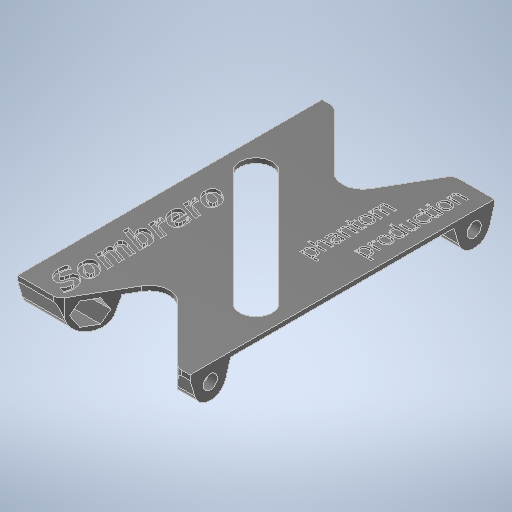
# Autodesk Inventor part: 3D_side-wall
Saved by Autodesk Inventor 2025 (Build 290162000, 162)
## iProperties
Created: 2024-06-30
Part Number: 3D_side-wall
Material: 一般
Document SubType Name: Modeling
Designer: 8326d
Density: 1 g/cm^3
Appearance: 滑らか - 黒
Author: 8326d
## iProperties of the stored document 3D_side-wall_3D プリント.ipt
Created: 2024-07-25
Part Number: 3D_side-wall_3D プリント
Material: 一般
Document SubType Name: Modeling
Designer: 8326d
Density: 1 g/cm^3
Appearance: 既定
Author: 8326d
Autodesk Inventor part; units mm, degrees
ref_plane "YZ Plane" through (0, 0, 0) normal (1, 0, 0) x (0, 1, 0)
ref_plane "XZ Plane" through (0, 0, 0) normal (0, 1, 0) x (-1, 0, 0)
ref_plane "XY Plane" through (0, 0, 0) normal (0, 0, 1) x (1, 0, 0)
sketch "スケッチ1" plane through (0, 0, 0) normal (0, 1, 0) x (-1, 0, 0)
  line L0 (-21.25, 37.5) -> (21.25, 37.5)
  line L1 (21.25, 37.5) -> (21.25, -37.5)
  line L2 (21.25, -37.5) -> (-21.25, -37.5)
  line L3 (-21.25, -37.5) -> (-21.25, 37.5)
  line L4 (-21.25, 37.5) -> (21.25, -37.5) construction
  line L5 (21.25, 37.5) -> (-21.25, -37.5) construction
  point P0 (0, 0)
  dimension "d0" = 42.5
  dimension "d1" = 75
  constraints: 12 end point, 2 midpoint, 2 parallel, 1 horizontal, 1 perpendicular
  measures "d0" distance of L1.end L2.end
  measures "d1" distance of L0.end L1.end
extrude "押し出し1" add sketch "スケッチ1" along normal mid plane 1.2
sketch "スケッチ2" plane through (21.25, 0.6, 37.5) normal (1, 0, 0) x (0, 0, -1)
  line L0 (0, 0) -> (75, 0) projected
  circle A0 centre (5, -4) radius 4
  line L1 (75, 0) -> (0, 0) projected
  circle A1 centre (70, -4) radius 4
  line L2 (75, -1.2) -> (0, -1.2) projected
  line L3 (1.1644, -5.135) -> (0, -1.2)
  line L4 (8.8356, -5.135) -> (10, -1.2)
  line L5 (66.1644, -5.135) -> (65, -1.2)
  line L6 (0, -1.2) -> (75, -1.2) projected
  line L7 (73.8356, -5.135) -> (75, -1.2)
  point P0 (37.5, -0.6)
  point P1 (67.1434, -1.2)
  point P2 (72.8566, -1.2)
  point P3 (2.1434, -1.2)
  point P4 (7.8566, -1.2)
  dimension "d4" = 8
  dimension "d5" = 8
  dimension "d6" = 5
  dimension "d7" = 5
  dimension "d8" = 5
  dimension "d9" = 5
  constraints: 8 end point, 6 tangent, 4 point on circle, 2 centre point, 2 point on line
  measures "d4" diameter of A0
  measures "d5" diameter of A1
  measures "d6" horizontal distance of L0.start A0.centre
  measures "d7" horizontal distance of L0.end A1.centre
  measures "d8" horizontal distance of A1.centre L5.end
  measures "d9" horizontal distance of A0.centre L4.end
extrude "押し出し2" add sketch "スケッチ2" against normal up to surface (42.5 mm away) contours A0 L2 | A1 L2 | L2 L4 A0 | A0 L2 | A0 L3 L2 | L2 L7 A1 | A1 L2 | A1 L5 L2
sketch "スケッチ3" plane through (0, 0.6, 0) normal (0, 1, 0) x (1, 0, 0)
  line L0 (14.1421, -14.1421) -> (-14.1421, 14.1421) construction
  line L1 (16.9706, -11.3137) -> (-11.3137, 16.9706)
  line L2 (-16.9706, 11.3137) -> (11.3137, -16.9706)
  arc A0 (11.3137, -16.9706) -> (16.9706, -11.3137) centre (14.1421, -14.1421) ccw
  arc A1 (-11.3137, 16.9706) -> (-16.9706, 11.3137) centre (-14.1421, 14.1421) ccw
  line L3 (-21.25, 37.5) -> (-21.25, -37.5) projected
  point P0 (0, 0)
  dimension "d12" = 45
  dimension "d13" = 40
  dimension "d14" = 4
  constraints: 8 end point, 4 point on circle, 4 tangent, 2 centre point, 1 midpoint, 1 parallel
  measures "d12" angle of L3 L0
  measures "d13" distance of L0.start L0.end
  measures "d14" radius of A1
extrude "押し出し3" cut sketch "スケッチ3" against normal through all
sketch "スケッチ4" plane through (0, 0.6, 0) normal (0, 1, 0) x (1, 0, 0)
  line L0 (7.2681, 1.9828) -> (7.2681, 38.4533) construction
  line L1 (7.2681, 38.4533) -> (15.699, 38.4533) construction
  line L2 (15.699, 38.4533) -> (15.699, 1.9828) construction
  line L3 (15.699, 1.9828) -> (7.2681, 1.9828) construction
  line L4 (-17.7945, -35.8694) -> (-17.7945, 8.3303) construction
  line L5 (-17.7945, 8.3303) -> (-9.6917, 8.3303) construction
  line L6 (-9.6917, 8.3303) -> (-9.6917, -35.8694) construction
  line L7 (-9.6917, -35.8694) -> (-17.7945, -35.8694) construction
  spline S0 degree 2 poles (-11.4201, -33.4285) (-11.4201, -34.119) (-11.6875, -35.072) (-11.882, -35.4512) knots 0 0 0 1 2 2 2
  line L8 (-11.882, -35.4512) -> (-13.3115, -34.965)
  line L9 (-13.3115, -34.965) -> (-13.3115, -34.8289)
  spline S1 degree 2 poles (-13.3115, -34.8289) (-12.9274, -34.508) (-12.5141, -33.5647) (-12.5141, -33.0541) knots 0 0 0 1 2 2 2
  spline S2 degree 2 poles (-12.5141, -33.0541) (-12.5141, -32.9229) (-12.5725, -32.4804) (-12.6308, -32.3345) knots 0 0 0 1 2 2 2
  spline S3 degree 2 poles (-12.6308, -32.3345) (-12.6989, -32.1546) (-12.9469, -31.8532) (-13.1462, -31.7851) knots 0 0 0 1 2 2 2
  spline S4 degree 2 poles (-13.1462, -31.7851) (-13.3747, -31.7073) (-13.6568, -31.965) (-13.72, -32.1887) knots 0 0 0 1 2 2 2
  spline S5 degree 2 poles (-13.72, -32.1887) (-13.8026, -32.4658) (-13.9436, -33.1125) (-14.0506, -33.3799) knots 0 0 0 1 2 2 2
  spline S6 degree 2 poles (-14.0506, -33.3799) (-14.2937, -33.9926) (-15.1252, -34.3183) (-15.7475, -34.1044) knots 0 0 0 1 2 2 2
  spline S7 degree 2 poles (-15.7475, -34.1044) (-16.5887, -33.8175) (-17.6341, -32.0379) (-17.6341, -30.9683) knots 0 0 0 1 2 2 2
  spline S8 degree 2 poles (-17.6341, -30.9683) (-17.6341, -30.4334) (-17.4153, -29.4512) (-17.2305, -29.0914) knots 0 0 0 1 2 2 2
  line L10 (-17.2305, -29.0914) -> (-15.8593, -29.5582)
  line L11 (-15.8593, -29.5582) -> (-15.8593, -29.6943)
  spline S9 degree 2 poles (-15.8593, -29.6943) (-16.1462, -29.9277) (-16.5401, -30.7543) (-16.5401, -31.2648) knots 0 0 0 1 2 2 2
  spline S10 degree 2 poles (-16.5401, -31.2648) (-16.5401, -31.4593) (-16.4817, -31.7948) (-16.4039, -31.9942) knots 0 0 0 1 2 2 2
  spline S11 degree 2 poles (-16.4039, -31.9942) (-16.3407, -32.1546) (-16.0879, -32.4464) (-15.9323, -32.4999) knots 0 0 0 1 2 2 2
  spline S12 degree 2 poles (-15.9323, -32.4999) (-15.6989, -32.5777) (-15.4315, -32.3443) (-15.3245, -31.9164) knots 0 0 0 1 2 2 2
  spline S13 degree 2 poles (-15.3245, -31.9164) (-15.2564, -31.6344) (-15.1252, -31.119) (-15.0133, -30.8418) knots 0 0 0 1 2 2 2
  spline S14 degree 2 poles (-15.0133, -30.8418) (-14.7848, -30.2924) (-14.0263, -29.9423) (-13.4039, -30.1563) knots 0 0 0 1 2 2 2
  spline S15 degree 2 poles (-13.4039, -30.1563) (-12.5093, -30.4577) (-11.4201, -32.2324) (-11.4201, -33.4285) knots 0 0 0 1 2 2 2
  spline S16 degree 2 poles (-13.788, -24.9926) (-12.6697, -25.3718) (-11.3861, -27.0298) (-11.3861, -28.1433) knots 0 0 0 1 2 2 2
  spline S17 degree 2 poles (-11.3861, -28.1433) (-11.3861, -29.2519) (-12.6697, -30.0444) (-13.788, -29.6652) knots 0 0 0 1 2 2 2
  spline S18 degree 2 poles (-13.788, -29.6652) (-14.9161, -29.2811) (-16.1948, -27.6182) (-16.1948, -26.5096) knots 0 0 0 1 2 2 2
  spline S19 degree 2 poles (-16.1948, -26.5096) (-16.1948, -25.401) (-14.9112, -24.6133) (-13.788, -24.9926) knots 0 0 0 1 2 2 2
  spline S20 degree 2 poles (-13.7783, -26.4415) (-14.1819, -26.3005) (-14.7216, -26.2519) (-14.882, -26.3151) knots 0 0 0 1 2 2 2
  spline S21 degree 2 poles (-14.882, -26.3151) (-15.0522, -26.3832) (-15.1835, -26.6506) (-15.1835, -26.8548) knots 0 0 0 1 2 2 2
  spline S22 degree 2 poles (-15.1835, -26.8548) (-15.1835, -27.0444) (-15.0668, -27.3896) (-14.9015, -27.5744) knots 0 0 0 1 2 2 2
  spline S23 degree 2 poles (-14.9015, -27.5744) (-14.7459, -27.7494) (-14.1965, -28.0801) (-13.7783, -28.2259) knots 0 0 0 1 2 2 2
  spline S24 degree 2 poles (-13.7783, -28.2259) (-13.365, -28.367) (-12.8545, -28.401) (-12.6989, -28.3426) knots 0 0 0 1 2 2 2
  spline S25 degree 2 poles (-12.6989, -28.3426) (-12.5433, -28.2843) (-12.3974, -27.9974) (-12.3974, -27.7883) knots 0 0 0 1 2 2 2
  spline S26 degree 2 poles (-12.3974, -27.7883) (-12.3974, -27.6182) (-12.5433, -27.2195) (-12.6892, -27.0639) knots 0 0 0 1 2 2 2
  spline S27 degree 2 poles (-12.6892, -27.0639) (-12.8593, -26.8791) (-13.3504, -26.5874) (-13.7783, -26.4415) knots 0 0 0 1 2 2 2
  line L12 (-11.5271, -19.6101) -> (-13.788, -18.8418)
  spline S28 degree 2 poles (-13.788, -18.8418) (-14.1235, -18.73) (-14.5806, -18.5987) (-14.7264, -18.6084) knots 0 0 0 1 2 2 2
  spline S29 degree 2 poles (-14.7264, -18.6084) (-14.8723, -18.6182) (-15.0036, -18.8272) (-15.0036, -19.0558) knots 0 0 0 1 2 2 2
  spline S30 degree 2 poles (-15.0036, -19.0558) (-15.0036, -19.2162) (-14.8626, -19.576) (-14.7313, -19.8046) knots 0 0 0 1 2 2 2
  line L13 (-14.7313, -19.8046) -> (-11.5271, -20.8937)
  line L14 (-11.5271, -20.8937) -> (-11.5271, -22.3135)
  line L15 (-11.5271, -22.3135) -> (-13.788, -21.5452)
  spline S31 degree 2 poles (-13.788, -21.5452) (-14.1187, -21.4334) (-14.5806, -21.3021) (-14.7264, -21.3167) knots 0 0 0 1 2 2 2
  spline S32 degree 2 poles (-14.7264, -21.3167) (-14.8723, -21.3264) (-15.0036, -21.5355) (-15.0036, -21.764) knots 0 0 0 1 2 2 2
  spline S33 degree 2 poles (-15.0036, -21.764) (-15.0036, -21.9342) (-14.8431, -22.3232) (-14.7313, -22.5177) knots 0 0 0 1 2 2 2
  line L16 (-14.7313, -22.5177) -> (-11.5271, -23.6068)
  line L17 (-11.5271, -23.6068) -> (-11.5271, -25.0169)
  line L18 (-11.5271, -25.0169) -> (-16.0538, -23.4804)
  line L19 (-16.0538, -23.4804) -> (-16.0538, -22.0704)
  line L20 (-16.0538, -22.0704) -> (-15.553, -22.2405)
  spline S34 degree 2 poles (-15.553, -22.2405) (-15.8448, -21.7932) (-16.1754, -21.0639) (-16.1754, -20.6846) knots 0 0 0 1 2 2 2
  spline S35 degree 2 poles (-16.1754, -20.6846) (-16.1754, -20.2665) (-15.7816, -19.7705) (-15.3877, -19.7365) knots 0 0 0 1 2 2 2
  spline S36 degree 2 poles (-15.3877, -19.7365) (-15.767, -19.2016) (-16.1754, -18.3459) (-16.1754, -17.9764) knots 0 0 0 1 2 2 2
  spline S37 degree 2 poles (-16.1754, -17.9764) (-16.1754, -17.6603) (-15.976, -17.2324) (-15.7718, -17.1255) knots 0 0 0 1 2 2 2
  spline S38 degree 2 poles (-15.7718, -17.1255) (-15.553, -17.0088) (-14.955, -17.0234) (-14.4736, -17.1887) knots 0 0 0 1 2 2 2
  line L21 (-14.4736, -17.1887) -> (-11.5271, -18.1903)
  line L22 (-11.5271, -18.1903) -> (-11.5271, -19.6101)
  spline S39 degree 2 poles (-13.8512, -11.9229) (-12.7718, -12.2875) (-11.4396, -13.8337) (-11.4396, -14.6457) knots 0 0 0 1 2 2 2
  spline S40 degree 2 poles (-11.4396, -14.6457) (-11.4396, -14.9812) (-11.5903, -15.4334) (-11.7508, -15.6571) knots 0 0 0 1 2 2 2
  line L23 (-11.7508, -15.6571) -> (-11.5271, -15.7932)
  line L24 (-11.5271, -15.7932) -> (-11.5271, -17.1449)
  line L25 (-11.5271, -17.1449) -> (-17.7945, -15.0153)
  line L26 (-17.7945, -15.0153) -> (-17.7945, -13.6052)
  line L27 (-17.7945, -13.6052) -> (-15.5773, -14.3588)
  spline S41 degree 2 poles (-15.5773, -14.3588) (-15.8448, -13.9553) (-16.1754, -13.2016) (-16.1754, -12.7786) knots 0 0 0 1 2 2 2
  spline S42 degree 2 poles (-16.1754, -12.7786) (-16.1754, -11.9909) (-14.9452, -11.5485) (-13.8512, -11.9229) knots 0 0 0 1 2 2 2
  spline S43 degree 2 poles (-13.8221, -13.3767) (-14.4979, -13.1433) (-15.0765, -13.3572) (-15.0765, -13.7851) knots 0 0 0 1 2 2 2
  spline S44 degree 2 poles (-15.0765, -13.7851) (-15.0765, -13.9747) (-14.955, -14.388) (-14.8334, -14.6117) knots 0 0 0 1 2 2 2
  line L28 (-14.8334, -14.6117) -> (-12.5676, -15.3799)
  spline S45 degree 2 poles (-12.5676, -15.3799) (-12.5093, -15.2584) (-12.4704, -14.9861) (-12.4704, -14.8451) knots 0 0 0 1 2 2 2
  spline S46 degree 2 poles (-12.4704, -14.8451) (-12.4704, -14.3345) (-13.1462, -13.6052) (-13.8221, -13.3767) knots 0 0 0 1 2 2 2
  line L29 (-14.7167, -7.8094) -> (-14.7167, -7.9261)
  spline S47 degree 2 poles (-14.7167, -7.9261) (-14.7459, -7.999) (-14.7751, -8.2956) (-14.7751, -8.4804) knots 0 0 0 1 2 2 2
  spline S48 degree 2 poles (-14.7751, -8.4804) (-14.7751, -8.6992) (-14.6438, -9.2341) (-14.5563, -9.4917) knots 0 0 0 1 2 2 2
  line L30 (-14.5563, -9.4917) -> (-11.5271, -10.5225)
  line L31 (-11.5271, -10.5225) -> (-11.5271, -11.9326)
  line L32 (-11.5271, -11.9326) -> (-16.0538, -10.3961)
  line L33 (-16.0538, -10.3961) -> (-16.0538, -8.9861)
  line L34 (-16.0538, -8.9861) -> (-15.4023, -9.2049)
  spline S49 degree 2 poles (-15.4023, -9.2049) (-15.4898, -9.0785) (-15.7621, -8.6457) (-15.8448, -8.4755) knots 0 0 0 1 2 2 2
  spline S50 degree 2 poles (-15.8448, -8.4755) (-15.9371, -8.2908) (-16.0684, -7.8386) (-16.0684, -7.6587) knots 0 0 0 1 2 2 2
  spline S51 degree 2 poles (-16.0684, -7.6587) (-16.0684, -7.5858) (-16.0587, -7.4204) (-16.0538, -7.3572) knots 0 0 0 1 2 2 2
  line L35 (-16.0538, -7.3572) -> (-14.7167, -7.8094)
  spline S52 degree 2 poles (-11.4055, -6.0785) (-11.4055, -7.3621) (-12.6308, -8.3102) (-13.7637, -7.9261) knots 0 0 0 1 2 2 2
  spline S53 degree 2 poles (-13.7637, -7.9261) (-14.8723, -7.5469) (-16.1948, -5.8256) (-16.1948, -4.6781) knots 0 0 0 1 2 2 2
  spline S54 degree 2 poles (-16.1948, -4.6781) (-16.1948, -3.6376) (-15.0717, -2.9715) (-14.0311, -3.3264) knots 0 0 0 1 2 2 2
  line L36 (-14.0311, -3.3264) -> (-13.5206, -3.5015)
  line L37 (-13.5206, -3.5015) -> (-13.5206, -6.5987)
  spline S55 degree 2 poles (-13.5206, -6.5987) (-13.2046, -6.6814) (-12.7864, -6.5987) (-12.66, -6.4577) knots 0 0 0 1 2 2 2
  spline S56 degree 2 poles (-12.66, -6.4577) (-12.5336, -6.3167) (-12.4266, -5.8694) (-12.4266, -5.5825) knots 0 0 0 1 2 2 2
  spline S57 degree 2 poles (-12.4266, -5.5825) (-12.4266, -5.3394) (-12.5336, -4.824) (-12.626, -4.5955) knots 0 0 0 1 2 2 2
  spline S58 degree 2 poles (-12.626, -4.5955) (-12.6989, -4.3961) (-12.8788, -4.0412) (-12.9469, -3.9245) knots 0 0 0 1 2 2 2
  line L38 (-12.9469, -3.9245) -> (-12.9469, -3.7786)
  line L39 (-12.9469, -3.7786) -> (-11.7799, -4.1725)
  spline S59 degree 2 poles (-11.7799, -4.1725) (-11.7119, -4.3718) (-11.5952, -4.6976) (-11.5368, -4.965) knots 0 0 0 1 2 2 2
  spline S60 degree 2 poles (-11.5368, -4.965) (-11.4736, -5.2178) (-11.4055, -5.7284) (-11.4055, -6.0785) knots 0 0 0 1 2 2 2
  spline S61 degree 2 poles (-14.3715, -4.6003) (-14.8188, -4.4593) (-15.2905, -4.6927) (-15.2905, -5.0963) knots 0 0 0 1 2 2 2
  spline S62 degree 2 poles (-15.2905, -5.0963) (-15.2905, -5.5096) (-14.7945, -6.1417) (-14.3715, -6.3118) knots 0 0 0 1 2 2 2
  line L40 (-14.3715, -6.3118) -> (-14.3715, -4.6003)
  line L41 (-14.7167, 0.6703) -> (-14.7167, 0.5536)
  spline S63 degree 2 poles (-14.7167, 0.5536) (-14.7459, 0.4807) (-14.7751, 0.1841) (-14.7751, -0.0007) knots 0 0 0 1 2 2 2
  spline S64 degree 2 poles (-14.7751, -0.0007) (-14.7751, -0.2195) (-14.6438, -0.7543) (-14.5563, -1.012) knots 0 0 0 1 2 2 2
  line L42 (-14.5563, -1.012) -> (-11.5271, -2.0428)
  line L43 (-11.5271, -2.0428) -> (-11.5271, -3.4529)
  line L44 (-11.5271, -3.4529) -> (-16.0538, -1.9164)
  line L45 (-16.0538, -1.9164) -> (-16.0538, -0.5063)
  line L46 (-16.0538, -0.5063) -> (-15.4023, -0.7251)
  spline S65 degree 2 poles (-15.4023, -0.7251) (-15.4898, -0.5987) (-15.7621, -0.166) (-15.8448, 0.0042) knots 0 0 0 1 2 2 2
  spline S66 degree 2 poles (-15.8448, 0.0042) (-15.9371, 0.189) (-16.0684, 0.6412) (-16.0684, 0.8211) knots 0 0 0 1 2 2 2
  spline S67 degree 2 poles (-16.0684, 0.8211) (-16.0684, 0.894) (-16.0587, 1.0593) (-16.0538, 1.1225) knots 0 0 0 1 2 2 2
  line L47 (-16.0538, 1.1225) -> (-14.7167, 0.6703)
  spline S68 degree 2 poles (-13.788, 5.236) (-12.6697, 4.8567) (-11.3861, 3.1987) (-11.3861, 2.0852) knots 0 0 0 1 2 2 2
  spline S69 degree 2 poles (-11.3861, 2.0852) (-11.3861, 0.9766) (-12.6697, 0.1841) (-13.788, 0.5634) knots 0 0 0 1 2 2 2
  spline S70 degree 2 poles (-13.788, 0.5634) (-14.9161, 0.9475) (-16.1948, 2.6104) (-16.1948, 3.7189) knots 0 0 0 1 2 2 2
  spline S71 degree 2 poles (-16.1948, 3.7189) (-16.1948, 4.8275) (-14.9112, 5.6152) (-13.788, 5.236) knots 0 0 0 1 2 2 2
  spline S72 degree 2 poles (-13.7783, 3.787) (-14.1819, 3.928) (-14.7216, 3.9766) (-14.882, 3.9134) knots 0 0 0 1 2 2 2
  spline S73 degree 2 poles (-14.882, 3.9134) (-15.0522, 3.8454) (-15.1835, 3.5779) (-15.1835, 3.3737) knots 0 0 0 1 2 2 2
  spline S74 degree 2 poles (-15.1835, 3.3737) (-15.1835, 3.1841) (-15.0668, 2.8389) (-14.9015, 2.6541) knots 0 0 0 1 2 2 2
  spline S75 degree 2 poles (-14.9015, 2.6541) (-14.7459, 2.4791) (-14.1965, 2.1484) (-13.7783, 2.0026) knots 0 0 0 1 2 2 2
  spline S76 degree 2 poles (-13.7783, 2.0026) (-13.365, 1.8616) (-12.8545, 1.8275) (-12.6989, 1.8859) knots 0 0 0 1 2 2 2
  spline S77 degree 2 poles (-12.6989, 1.8859) (-12.5433, 1.9442) (-12.3974, 2.2311) (-12.3974, 2.4402) knots 0 0 0 1 2 2 2
  spline S78 degree 2 poles (-12.3974, 2.4402) (-12.3974, 2.6104) (-12.5433, 3.0091) (-12.6892, 3.1647) knots 0 0 0 1 2 2 2
  spline S79 degree 2 poles (-12.6892, 3.1647) (-12.8593, 3.3494) (-13.3504, 3.6412) (-13.7783, 3.787) knots 0 0 0 1 2 2 2
  spline S80 degree 2 poles (9.8645, 4.8645) (10.6165, 4.8645) (11.5047, 4.1481) (11.5047, 3.6003) knots 0 0 0 1 2 2 2
  spline S81 degree 2 poles (11.5047, 3.6003) (11.5047, 3.3767) (11.401, 3.0331) (11.294, 2.8548) knots 0 0 0 1 2 2 2
  line L48 (11.294, 2.8548) -> (12.5517, 2.8548)
  line L49 (12.5517, 2.8548) -> (12.5517, 2.3491)
  line L50 (12.5517, 2.3491) -> (8.4447, 2.3491)
  line L51 (8.4447, 2.3491) -> (8.4447, 2.8548)
  line L52 (8.4447, 2.8548) -> (8.7592, 2.8548)
  spline S82 degree 2 poles (8.7592, 2.8548) (8.5874, 3.0428) (8.3605, 3.5031) (8.3605, 3.7721) knots 0 0 0 1 2 2 2
  spline S83 degree 2 poles (8.3605, 3.7721) (8.3605, 4.2875) (9.1773, 4.8645) (9.8645, 4.8645) knots 0 0 0 1 2 2 2
  spline S84 degree 2 poles (9.9229, 4.3426) (9.4075, 4.3426) (8.8402, 4.0152) (8.8402, 3.649) knots 0 0 0 1 2 2 2
  spline S85 degree 2 poles (8.8402, 3.649) (8.8402, 3.435) (9.0315, 3.0331) (9.1806, 2.8548) knots 0 0 0 1 2 2 2
  line L53 (9.1806, 2.8548) -> (10.8856, 2.8548)
  spline S86 degree 2 poles (10.8856, 2.8548) (10.9796, 3.0525) (11.0509, 3.3345) (11.0509, 3.5161) knots 0 0 0 1 2 2 2
  spline S87 degree 2 poles (11.0509, 3.5161) (11.0509, 3.9083) (10.4739, 4.3426) (9.9229, 4.3426) knots 0 0 0 1 2 2 2
  line L54 (11.4464, 7.7462) -> (11.4464, 7.2405)
  line L55 (11.4464, 7.2405) -> (9.7349, 7.2405)
  spline S88 degree 2 poles (9.7349, 7.2405) (9.5274, 7.2405) (9.1708, 7.2016) (9.0639, 7.1433) knots 0 0 0 1 2 2 2
  spline S89 degree 2 poles (9.0639, 7.1433) (8.9504, 7.0817) (8.8402, 6.8613) (8.8402, 6.6733) knots 0 0 0 1 2 2 2
  spline S90 degree 2 poles (8.8402, 6.6733) (8.8402, 6.4853) (9.0412, 6.0866) (9.2033, 5.8953) knots 0 0 0 1 2 2 2
  line L56 (9.2033, 5.8953) -> (11.4464, 5.8953)
  line L57 (11.4464, 5.8953) -> (11.4464, 5.3896)
  line L58 (11.4464, 5.3896) -> (7.2681, 5.3896)
  line L59 (7.2681, 5.3896) -> (7.2681, 5.8953)
  line L60 (7.2681, 5.8953) -> (8.7786, 5.8953)
  spline S91 degree 2 poles (8.7786, 5.8953) (8.5744, 6.1222) (8.3605, 6.5598) (8.3605, 6.8062) knots 0 0 0 1 2 2 2
  spline S92 degree 2 poles (8.3605, 6.8062) (8.3605, 7.247) (8.9439, 7.7462) (9.4982, 7.7462) knots 0 0 0 1 2 2 2
  line L61 (9.4982, 7.7462) -> (11.4464, 7.7462)
  spline S93 degree 2 poles (11.1287, 10.1287) (11.1741, 10.0671) (11.3362, 9.8596) (11.3848, 9.7624) knots 0 0 0 1 2 2 2
  spline S94 degree 2 poles (11.3848, 9.7624) (11.4561, 9.6295) (11.5306, 9.3799) (11.5306, 9.153) knots 0 0 0 1 2 2 2
  spline S95 degree 2 poles (11.5306, 9.153) (11.5306, 8.9682) (11.3913, 8.6344) (11.2648, 8.5079) knots 0 0 0 1 2 2 2
  spline S96 degree 2 poles (11.2648, 8.5079) (11.1417, 8.388) (10.7786, 8.2421) (10.5776, 8.2421) knots 0 0 0 1 2 2 2
  spline S97 degree 2 poles (10.5776, 8.2421) (10.2665, 8.2421) (9.8256, 8.5047) (9.6992, 8.79) knots 0 0 0 1 2 2 2
  spline S98 degree 2 poles (9.6992, 8.79) (9.5825, 9.0428) (9.495, 9.73) (9.4723, 10.1287) knots 0 0 0 1 2 2 2
  line L62 (9.4723, 10.1287) -> (9.3751, 10.1287)
  spline S99 degree 2 poles (9.3751, 10.1287) (9.2, 10.1287) (8.9828, 10.0217) (8.9212, 9.9245) knots 0 0 0 1 2 2 2
  spline S100 degree 2 poles (8.9212, 9.9245) (8.8597, 9.8272) (8.8208, 9.5485) (8.8208, 9.3994) knots 0 0 0 1 2 2 2
  spline S101 degree 2 poles (8.8208, 9.3994) (8.8208, 9.2243) (8.9245, 8.7511) (9.025, 8.5144) knots 0 0 0 1 2 2 2
  line L63 (9.025, 8.5144) -> (9.025, 8.4853)
  line L64 (9.025, 8.4853) -> (8.5096, 8.4853)
  spline S102 degree 2 poles (8.5096, 8.4853) (8.4707, 8.6246) (8.3734, 9.1465) (8.3734, 9.4026) knots 0 0 0 1 2 2 2
  spline S103 degree 2 poles (8.3734, 9.4026) (8.3734, 9.7138) (8.4707, 10.1384) (8.5971, 10.307) knots 0 0 0 1 2 2 2
  spline S104 degree 2 poles (8.5971, 10.307) (8.7203, 10.4723) (9.1125, 10.6344) (9.3945, 10.6344) knots 0 0 0 1 2 2 2
  line L65 (9.3945, 10.6344) -> (11.4464, 10.6344)
  line L66 (11.4464, 10.6344) -> (11.4464, 10.1287)
  line L67 (11.4464, 10.1287) -> (11.1287, 10.1287)
  line L68 (10.7073, 10.1287) -> (9.8742, 10.1287)
  spline S105 degree 2 poles (9.8742, 10.1287) (9.8905, 9.9472) (9.9456, 9.3994) (9.9974, 9.2276) knots 0 0 0 1 2 2 2
  spline S106 degree 2 poles (9.9974, 9.2276) (10.059, 9.0266) (10.3151, 8.764) (10.542, 8.764) knots 0 0 0 1 2 2 2
  spline S107 degree 2 poles (10.542, 8.764) (10.8013, 8.764) (11.0639, 9.0558) (11.0639, 9.3345) knots 0 0 0 1 2 2 2
  spline S108 degree 2 poles (11.0639, 9.3345) (11.0639, 9.5712) (10.8597, 9.9601) (10.7073, 10.1287) knots 0 0 0 1 2 2 2
  line L69 (11.4464, 13.7008) -> (11.4464, 13.1951)
  line L70 (11.4464, 13.1951) -> (9.7349, 13.1951)
  spline S109 degree 2 poles (9.7349, 13.1951) (9.5274, 13.1951) (9.1708, 13.1562) (9.0639, 13.0979) knots 0 0 0 1 2 2 2
  spline S110 degree 2 poles (9.0639, 13.0979) (8.9504, 13.0363) (8.8402, 12.8159) (8.8402, 12.6279) knots 0 0 0 1 2 2 2
  spline S111 degree 2 poles (8.8402, 12.6279) (8.8402, 12.4399) (9.0412, 12.0412) (9.2033, 11.8499) knots 0 0 0 1 2 2 2
  line L71 (9.2033, 11.8499) -> (11.4464, 11.8499)
  line L72 (11.4464, 11.8499) -> (11.4464, 11.3443)
  line L73 (11.4464, 11.3443) -> (8.4447, 11.3443)
  line L74 (8.4447, 11.3443) -> (8.4447, 11.8499)
  line L75 (8.4447, 11.8499) -> (8.7786, 11.8499)
  spline S112 degree 2 poles (8.7786, 11.8499) (8.5744, 12.0768) (8.3605, 12.5144) (8.3605, 12.7608) knots 0 0 0 1 2 2 2
  spline S113 degree 2 poles (8.3605, 12.7608) (8.3605, 13.2016) (8.9439, 13.7008) (9.4982, 13.7008) knots 0 0 0 1 2 2 2
  line L76 (9.4982, 13.7008) -> (11.4464, 13.7008)
  spline S114 degree 2 poles (11.5047, 15.3183) (11.5047, 14.9067) (11.0347, 14.4431) (10.5258, 14.4431) knots 0 0 0 1 2 2 2
  line L77 (10.5258, 14.4431) -> (8.8629, 14.4431)
  line L78 (8.8629, 14.4431) -> (8.8629, 14.1028)
  line L79 (8.8629, 14.1028) -> (8.4447, 14.1028)
  line L80 (8.4447, 14.1028) -> (8.4447, 14.4431)
  line L81 (8.4447, 14.4431) -> (7.5825, 14.4431)
  line L82 (7.5825, 14.4431) -> (7.5825, 14.9488)
  line L83 (7.5825, 14.9488) -> (8.4447, 14.9488)
  line L84 (8.4447, 14.9488) -> (8.4447, 15.8791)
  line L85 (8.4447, 15.8791) -> (8.8629, 15.8791)
  line L86 (8.8629, 15.8791) -> (8.8629, 14.9488)
  line L87 (8.8629, 14.9488) -> (10.2924, 14.9488)
  spline S115 degree 2 poles (10.2924, 14.9488) (10.5193, 14.9488) (10.7689, 14.965) (10.8759, 15.0201) knots 0 0 0 1 2 2 2
  spline S116 degree 2 poles (10.8759, 15.0201) (10.9699, 15.0655) (11.0639, 15.2697) (11.0639, 15.4447) knots 0 0 0 1 2 2 2
  spline S117 degree 2 poles (11.0639, 15.4447) (11.0639, 15.5679) (10.9893, 15.7981) (10.9666, 15.8499) knots 0 0 0 1 2 2 2
  line L88 (10.9666, 15.8499) -> (10.9666, 15.8791)
  line L89 (10.9666, 15.8791) -> (11.4204, 15.8791)
  spline S118 degree 2 poles (11.4204, 15.8791) (11.4593, 15.7365) (11.5047, 15.4447) (11.5047, 15.3183) knots 0 0 0 1 2 2 2
  spline S119 degree 2 poles (9.9456, 18.7186) (10.7041, 18.7186) (11.5306, 17.9893) (11.5306, 17.3799) knots 0 0 0 1 2 2 2
  spline S120 degree 2 poles (11.5306, 17.3799) (11.5306, 16.7543) (10.6781, 16.0379) (9.9456, 16.0379) knots 0 0 0 1 2 2 2
  spline S121 degree 2 poles (9.9456, 16.0379) (9.1935, 16.0379) (8.3605, 16.777) (8.3605, 17.3799) knots 0 0 0 1 2 2 2
  spline S122 degree 2 poles (8.3605, 17.3799) (8.3605, 17.9893) (9.1903, 18.7186) (9.9456, 18.7186) knots 0 0 0 1 2 2 2
  spline S123 degree 2 poles (9.9456, 18.1968) (9.3621, 18.1968) (8.7948, 17.7721) (8.7948, 17.3799) knots 0 0 0 1 2 2 2
  spline S124 degree 2 poles (8.7948, 17.3799) (8.7948, 16.9877) (9.3621, 16.5598) (9.9456, 16.5598) knots 0 0 0 1 2 2 2
  spline S125 degree 2 poles (9.9456, 16.5598) (10.5128, 16.5598) (11.0963, 16.9877) (11.0963, 17.3799) knots 0 0 0 1 2 2 2
  spline S126 degree 2 poles (11.0963, 17.3799) (11.0963, 17.7689) (10.5225, 18.1968) (9.9456, 18.1968) knots 0 0 0 1 2 2 2
  line L90 (11.4464, 22.6408) -> (9.7089, 22.6408)
  spline S127 degree 2 poles (9.7089, 22.6408) (9.5015, 22.6408) (9.1482, 22.6084) (9.0509, 22.5566) knots 0 0 0 1 2 2 2
  spline S128 degree 2 poles (9.0509, 22.5566) (8.9439, 22.5047) (8.8402, 22.307) (8.8402, 22.1352) knots 0 0 0 1 2 2 2
  spline S129 degree 2 poles (8.8402, 22.1352) (8.8402, 21.9796) (9.0315, 21.623) (9.213, 21.435) knots 0 0 0 1 2 2 2
  spline S130 degree 2 poles (9.213, 21.435) (9.2584, 21.4383) (9.3848, 21.4447) (9.4691, 21.4447) knots 0 0 0 1 2 2 2
  line L91 (9.4691, 21.4447) -> (11.4464, 21.4447)
  line L92 (11.4464, 21.4447) -> (11.4464, 20.9391)
  line L93 (11.4464, 20.9391) -> (9.7089, 20.9391)
  spline S131 degree 2 poles (9.7089, 20.9391) (9.5015, 20.9391) (9.1482, 20.9067) (9.0509, 20.8548) knots 0 0 0 1 2 2 2
  spline S132 degree 2 poles (9.0509, 20.8548) (8.9439, 20.8029) (8.8402, 20.6052) (8.8402, 20.4334) knots 0 0 0 1 2 2 2
  spline S133 degree 2 poles (8.8402, 20.4334) (8.8402, 20.2713) (9.0444, 19.9115) (9.2033, 19.743) knots 0 0 0 1 2 2 2
  line L94 (9.2033, 19.743) -> (11.4464, 19.743)
  line L95 (11.4464, 19.743) -> (11.4464, 19.2373)
  line L96 (11.4464, 19.2373) -> (8.4447, 19.2373)
  line L97 (8.4447, 19.2373) -> (8.4447, 19.743)
  line L98 (8.4447, 19.743) -> (8.7754, 19.743)
  spline S134 degree 2 poles (8.7754, 19.743) (8.5776, 19.9407) (8.3605, 20.3297) (8.3605, 20.5631) knots 0 0 0 1 2 2 2
  spline S135 degree 2 poles (8.3605, 20.5631) (8.3605, 20.8289) (8.6036, 21.2405) (8.8791, 21.3475) knots 0 0 0 1 2 2 2
  spline S136 degree 2 poles (8.8791, 21.3475) (8.623, 21.5776) (8.3605, 22.012) (8.3605, 22.2648) knots 0 0 0 1 2 2 2
  spline S137 degree 2 poles (8.3605, 22.2648) (8.3605, 22.4593) (8.4804, 22.777) (8.6165, 22.8937) knots 0 0 0 1 2 2 2
  spline S138 degree 2 poles (8.6165, 22.8937) (8.7527, 23.0136) (9.1611, 23.1465) (9.4691, 23.1465) knots 0 0 0 1 2 2 2
  line L99 (9.4691, 23.1465) -> (11.4464, 23.1465)
  line L100 (11.4464, 23.1465) -> (11.4464, 22.6408)
  spline S139 degree 2 poles (16.4504, 11.7365) (17.2024, 11.7365) (18.0906, 11.0201) (18.0906, 10.4723) knots 0 0 0 1 2 2 2
  spline S140 degree 2 poles (18.0906, 10.4723) (18.0906, 10.2486) (17.9869, 9.905) (17.8799, 9.7267) knots 0 0 0 1 2 2 2
  line L101 (17.8799, 9.7267) -> (19.1376, 9.7267)
  line L102 (19.1376, 9.7267) -> (19.1376, 9.2211)
  line L103 (19.1376, 9.2211) -> (15.0306, 9.2211)
  line L104 (15.0306, 9.2211) -> (15.0306, 9.7267)
  line L105 (15.0306, 9.7267) -> (15.3451, 9.7267)
  spline S141 degree 2 poles (15.3451, 9.7267) (15.1733, 9.9148) (14.9464, 10.375) (14.9464, 10.6441) knots 0 0 0 1 2 2 2
  spline S142 degree 2 poles (14.9464, 10.6441) (14.9464, 11.1595) (15.7632, 11.7365) (16.4504, 11.7365) knots 0 0 0 1 2 2 2
  spline S143 degree 2 poles (16.5088, 11.2146) (15.9934, 11.2146) (15.4261, 10.8872) (15.4261, 10.5209) knots 0 0 0 1 2 2 2
  spline S144 degree 2 poles (15.4261, 10.5209) (15.4261, 10.307) (15.6174, 9.905) (15.7665, 9.7267) knots 0 0 0 1 2 2 2
  line L106 (15.7665, 9.7267) -> (17.4715, 9.7267)
  spline S145 degree 2 poles (17.4715, 9.7267) (17.5655, 9.9245) (17.6368, 10.2065) (17.6368, 10.388) knots 0 0 0 1 2 2 2
  spline S146 degree 2 poles (17.6368, 10.388) (17.6368, 10.7802) (17.0598, 11.2146) (16.5088, 11.2146) knots 0 0 0 1 2 2 2
  line L107 (15.572, 13.8532) -> (15.572, 13.8272)
  spline S147 degree 2 poles (15.572, 13.8272) (15.5558, 13.7689) (15.5493, 13.6425) (15.5493, 13.5549) knots 0 0 0 1 2 2 2
  spline S148 degree 2 poles (15.5493, 13.5549) (15.5493, 13.3507) (15.7276, 12.9488) (15.9026, 12.7673) knots 0 0 0 1 2 2 2
  line L108 (15.9026, 12.7673) -> (18.0323, 12.7673)
  line L109 (18.0323, 12.7673) -> (18.0323, 12.2616)
  line L110 (18.0323, 12.2616) -> (15.0306, 12.2616)
  line L111 (15.0306, 12.2616) -> (15.0306, 12.7673)
  line L112 (15.0306, 12.7673) -> (15.478, 12.7673)
  spline S149 degree 2 poles (15.478, 12.7673) (15.2316, 13.0428) (15.0306, 13.4545) (15.0306, 13.649) knots 0 0 0 1 2 2 2
  spline S150 degree 2 poles (15.0306, 13.649) (15.0306, 13.7267) (15.0371, 13.8045) (15.0468, 13.8532) knots 0 0 0 1 2 2 2
  line L113 (15.0468, 13.8532) -> (15.572, 13.8532)
  spline S151 degree 2 poles (16.5315, 16.7122) (17.29, 16.7122) (18.1165, 15.9828) (18.1165, 15.3734) knots 0 0 0 1 2 2 2
  spline S152 degree 2 poles (18.1165, 15.3734) (18.1165, 14.7478) (17.264, 14.0314) (16.5315, 14.0314) knots 0 0 0 1 2 2 2
  spline S153 degree 2 poles (16.5315, 14.0314) (15.7794, 14.0314) (14.9464, 14.7705) (14.9464, 15.3734) knots 0 0 0 1 2 2 2
  spline S154 degree 2 poles (14.9464, 15.3734) (14.9464, 15.9828) (15.7762, 16.7122) (16.5315, 16.7122) knots 0 0 0 1 2 2 2
  spline S155 degree 2 poles (16.5315, 16.1903) (15.948, 16.1903) (15.3807, 15.7656) (15.3807, 15.3734) knots 0 0 0 1 2 2 2
  spline S156 degree 2 poles (15.3807, 15.3734) (15.3807, 14.9812) (15.948, 14.5533) (16.5315, 14.5533) knots 0 0 0 1 2 2 2
  spline S157 degree 2 poles (16.5315, 14.5533) (17.0987, 14.5533) (17.6822, 14.9812) (17.6822, 15.3734) knots 0 0 0 1 2 2 2
  spline S158 degree 2 poles (17.6822, 15.3734) (17.6822, 15.7624) (17.1084, 16.1903) (16.5315, 16.1903) knots 0 0 0 1 2 2 2
  line L114 (18.0323, 19.5387) -> (18.0323, 19.0331)
  line L115 (18.0323, 19.0331) -> (17.7276, 19.0331)
  spline S159 degree 2 poles (17.7276, 19.0331) (17.8248, 18.9164) (17.9545, 18.7446) (18.0096, 18.6279) knots 0 0 0 1 2 2 2
  spline S160 degree 2 poles (18.0096, 18.6279) (18.0614, 18.5209) (18.1165, 18.2908) (18.1165, 18.1384) knots 0 0 0 1 2 2 2
  spline S161 degree 2 poles (18.1165, 18.1384) (18.1165, 17.8921) (17.9123, 17.4772) (17.7146, 17.3313) knots 0 0 0 1 2 2 2
  spline S162 degree 2 poles (17.7146, 17.3313) (17.5169, 17.1854) (16.9334, 17.0233) (16.5541, 17.0233) knots 0 0 0 1 2 2 2
  spline S163 degree 2 poles (16.5541, 17.0233) (16.1587, 17.0233) (15.5817, 17.2276) (15.3645, 17.4058) knots 0 0 0 1 2 2 2
  spline S164 degree 2 poles (15.3645, 17.4058) (15.17, 17.5712) (14.9464, 18.0347) (14.9464, 18.2908) knots 0 0 0 1 2 2 2
  spline S165 degree 2 poles (14.9464, 18.2908) (14.9464, 18.5144) (15.0468, 18.8483) (15.1506, 19.0331) knots 0 0 0 1 2 2 2
  line L116 (15.1506, 19.0331) -> (13.854, 19.0331)
  line L117 (13.854, 19.0331) -> (13.854, 19.5387)
  line L118 (13.854, 19.5387) -> (18.0323, 19.5387)
  line L119 (17.3029, 19.0331) -> (15.5687, 19.0331)
  spline S166 degree 2 poles (15.5687, 19.0331) (15.478, 18.8451) (15.4099, 18.5468) (15.4099, 18.375) knots 0 0 0 1 2 2 2
  spline S167 degree 2 poles (15.4099, 18.375) (15.4099, 17.9861) (15.9934, 17.5452) (16.5444, 17.5452) knots 0 0 0 1 2 2 2
  spline S168 degree 2 poles (16.5444, 17.5452) (17.076, 17.5452) (17.6368, 17.8823) (17.6368, 18.2551) knots 0 0 0 1 2 2 2
  spline S169 degree 2 poles (17.6368, 18.2551) (17.6368, 18.4528) (17.4553, 18.8548) (17.3029, 19.0331) knots 0 0 0 1 2 2 2
  line L120 (18.0323, 22.6052) -> (18.0323, 22.0995)
  line L121 (18.0323, 22.0995) -> (17.7016, 22.0995)
  spline S170 degree 2 poles (17.7016, 22.0995) (17.9058, 21.8661) (18.1165, 21.448) (18.1165, 21.1887) knots 0 0 0 1 2 2 2
  spline S171 degree 2 poles (18.1165, 21.1887) (18.1165, 20.9942) (17.9869, 20.6473) (17.8475, 20.5209) knots 0 0 0 1 2 2 2
  spline S172 degree 2 poles (17.8475, 20.5209) (17.7081, 20.3913) (17.2835, 20.2486) (16.9788, 20.2486) knots 0 0 0 1 2 2 2
  line L122 (16.9788, 20.2486) -> (15.0306, 20.2486)
  line L123 (15.0306, 20.2486) -> (15.0306, 20.7543)
  line L124 (15.0306, 20.7543) -> (16.7421, 20.7543)
  spline S173 degree 2 poles (16.7421, 20.7543) (16.982, 20.7543) (17.2964, 20.79) (17.4131, 20.8515) knots 0 0 0 1 2 2 2
  spline S174 degree 2 poles (17.4131, 20.8515) (17.5298, 20.9131) (17.6368, 21.1238) (17.6368, 21.3216) knots 0 0 0 1 2 2 2
  spline S175 degree 2 poles (17.6368, 21.3216) (17.6368, 21.5063) (17.4261, 21.9245) (17.2738, 22.0995) knots 0 0 0 1 2 2 2
  line L125 (17.2738, 22.0995) -> (15.0306, 22.0995)
  line L126 (15.0306, 22.0995) -> (15.0306, 22.6052)
  line L127 (15.0306, 22.6052) -> (18.0323, 22.6052)
  spline S176 degree 2 poles (18.1003, 24.5306) (18.1003, 24.2195) (17.9091, 23.7041) (17.7146, 23.5193) knots 0 0 0 1 2 2 2
  spline S177 degree 2 poles (17.7146, 23.5193) (17.5233, 23.3345) (16.9334, 23.1303) (16.5379, 23.1303) knots 0 0 0 1 2 2 2
  spline S178 degree 2 poles (16.5379, 23.1303) (16.1425, 23.1303) (15.5655, 23.341) (15.371, 23.5193) knots 0 0 0 1 2 2 2
  spline S179 degree 2 poles (15.371, 23.5193) (15.1733, 23.6976) (14.9626, 24.2259) (14.9626, 24.5306) knots 0 0 0 1 2 2 2
  spline S180 degree 2 poles (14.9626, 24.5306) (14.9626, 24.777) (15.102, 25.2373) (15.1927, 25.4156) knots 0 0 0 1 2 2 2
  line L128 (15.1927, 25.4156) -> (15.76, 25.4156)
  line L129 (15.76, 25.4156) -> (15.76, 25.3864)
  spline S181 degree 2 poles (15.76, 25.3864) (15.7146, 25.3313) (15.5979, 25.1627) (15.5363, 25.0428) knots 0 0 0 1 2 2 2
  spline S182 degree 2 poles (15.5363, 25.0428) (15.4844, 24.9358) (15.4034, 24.6506) (15.4034, 24.5209) knots 0 0 0 1 2 2 2
  spline S183 degree 2 poles (15.4034, 24.5209) (15.4034, 24.1287) (15.9966, 23.6522) (16.5379, 23.6522) knots 0 0 0 1 2 2 2
  spline S184 degree 2 poles (16.5379, 23.6522) (17.0663, 23.6522) (17.6595, 24.1125) (17.6595, 24.5209) knots 0 0 0 1 2 2 2
  spline S185 degree 2 poles (17.6595, 24.5209) (17.6595, 24.7673) (17.4553, 25.2146) (17.2964, 25.3864) knots 0 0 0 1 2 2 2
  line L130 (17.2964, 25.3864) -> (17.2964, 25.4156)
  line L131 (17.2964, 25.4156) -> (17.8637, 25.4156)
  spline S186 degree 2 poles (17.8637, 25.4156) (17.8994, 25.341) (17.9998, 25.1141) (18.0225, 25.0233) knots 0 0 0 1 2 2 2
  spline S187 degree 2 poles (18.0225, 25.0233) (18.0614, 24.8937) (18.1003, 24.6895) (18.1003, 24.5306) knots 0 0 0 1 2 2 2
  spline S188 degree 2 poles (18.0906, 26.7835) (18.0906, 26.3718) (17.6206, 25.9083) (17.1117, 25.9083) knots 0 0 0 1 2 2 2
  line L132 (17.1117, 25.9083) -> (15.4488, 25.9083)
  line L133 (15.4488, 25.9083) -> (15.4488, 25.5679)
  line L134 (15.4488, 25.5679) -> (15.0306, 25.5679)
  line L135 (15.0306, 25.5679) -> (15.0306, 25.9083)
  line L136 (15.0306, 25.9083) -> (14.1684, 25.9083)
  line L137 (14.1684, 25.9083) -> (14.1684, 26.4139)
  line L138 (14.1684, 26.4139) -> (15.0306, 26.4139)
  line L139 (15.0306, 26.4139) -> (15.0306, 27.3443)
  line L140 (15.0306, 27.3443) -> (15.4488, 27.3443)
  line L141 (15.4488, 27.3443) -> (15.4488, 26.4139)
  line L142 (15.4488, 26.4139) -> (16.8783, 26.4139)
  spline S189 degree 2 poles (16.8783, 26.4139) (17.1052, 26.4139) (17.3548, 26.4302) (17.4618, 26.4853) knots 0 0 0 1 2 2 2
  spline S190 degree 2 poles (17.4618, 26.4853) (17.5558, 26.5306) (17.6498, 26.7349) (17.6498, 26.9099) knots 0 0 0 1 2 2 2
  spline S191 degree 2 poles (17.6498, 26.9099) (17.6498, 27.0331) (17.5752, 27.2632) (17.5525, 27.3151) knots 0 0 0 1 2 2 2
  line L143 (17.5525, 27.3151) -> (17.5525, 27.3443)
  line L144 (17.5525, 27.3443) -> (18.0063, 27.3443)
  spline S192 degree 2 poles (18.0063, 27.3443) (18.0452, 27.2016) (18.0906, 26.9099) (18.0906, 26.7835) knots 0 0 0 1 2 2 2
  line L145 (18.0323, 28.2324) -> (18.0323, 27.7267)
  line L146 (18.0323, 27.7267) -> (15.0306, 27.7267)
  line L147 (15.0306, 27.7267) -> (15.0306, 28.2324)
  line L148 (15.0306, 28.2324) -> (18.0323, 28.2324)
  line L149 (14.5315, 28.2681) -> (14.5315, 27.6943)
  line L150 (14.5315, 27.6943) -> (14.0063, 27.6943)
  line L151 (14.0063, 27.6943) -> (14.0063, 28.2681)
  line L152 (14.0063, 28.2681) -> (14.5315, 28.2681)
  spline S193 degree 2 poles (16.5315, 31.4415) (17.29, 31.4415) (18.1165, 30.7122) (18.1165, 30.1028) knots 0 0 0 1 2 2 2
  spline S194 degree 2 poles (18.1165, 30.1028) (18.1165, 29.4772) (17.264, 28.7608) (16.5315, 28.7608) knots 0 0 0 1 2 2 2
  spline S195 degree 2 poles (16.5315, 28.7608) (15.7794, 28.7608) (14.9464, 29.4998) (14.9464, 30.1028) knots 0 0 0 1 2 2 2
  spline S196 degree 2 poles (14.9464, 30.1028) (14.9464, 30.7122) (15.7762, 31.4415) (16.5315, 31.4415) knots 0 0 0 1 2 2 2
  spline S197 degree 2 poles (16.5315, 30.9196) (15.948, 30.9196) (15.3807, 30.495) (15.3807, 30.1028) knots 0 0 0 1 2 2 2
  spline S198 degree 2 poles (15.3807, 30.1028) (15.3807, 29.7105) (15.948, 29.2827) (16.5315, 29.2827) knots 0 0 0 1 2 2 2
  spline S199 degree 2 poles (16.5315, 29.2827) (17.0987, 29.2827) (17.6822, 29.7105) (17.6822, 30.1028) knots 0 0 0 1 2 2 2
  spline S200 degree 2 poles (17.6822, 30.1028) (17.6822, 30.4917) (17.1084, 30.9196) (16.5315, 30.9196) knots 0 0 0 1 2 2 2
  line L153 (18.0323, 34.3167) -> (18.0323, 33.811)
  line L154 (18.0323, 33.811) -> (16.3208, 33.811)
  spline S201 degree 2 poles (16.3208, 33.811) (16.1133, 33.811) (15.7567, 33.7721) (15.6498, 33.7138) knots 0 0 0 1 2 2 2
  spline S202 degree 2 poles (15.6498, 33.7138) (15.5363, 33.6522) (15.4261, 33.4318) (15.4261, 33.2438) knots 0 0 0 1 2 2 2
  spline S203 degree 2 poles (15.4261, 33.2438) (15.4261, 33.0558) (15.6271, 32.6571) (15.7891, 32.4658) knots 0 0 0 1 2 2 2
  line L155 (15.7891, 32.4658) -> (18.0323, 32.4658)
  line L156 (18.0323, 32.4658) -> (18.0323, 31.9601)
  line L157 (18.0323, 31.9601) -> (15.0306, 31.9601)
  line L158 (15.0306, 31.9601) -> (15.0306, 32.4658)
  line L159 (15.0306, 32.4658) -> (15.3645, 32.4658)
  spline S204 degree 2 poles (15.3645, 32.4658) (15.1603, 32.6927) (14.9464, 33.1303) (14.9464, 33.3767) knots 0 0 0 1 2 2 2
  spline S205 degree 2 poles (14.9464, 33.3767) (14.9464, 33.8175) (15.5298, 34.3167) (16.0841, 34.3167) knots 0 0 0 1 2 2 2
  line L160 (16.0841, 34.3167) -> (18.0323, 34.3167)
  point P0 (0, 0)
  constraints: 4 other
extrude "押し出し4" cut sketch "スケッチ4" against normal blind 0.8
sketch "スケッチ5" plane through (-21.25, 0.6, -37.5) normal (-1, 0, 0) x (0, 0, 1)
  arc A0 (66.1644, -5.135) -> (73.8356, -5.135) centre (70, -4) ccw projected
  arc A1 (1.1644, -5.135) -> (8.8356, -5.135) centre (5, -4) ccw projected
  point P0 (37.5, -0.6)
hole "穴1" at (-21.25, -3.4, -32.5) at (-21.25, -3.4, 32.5) direction (1, 0, 0) diameter 3.5 end through all
sketch "スケッチ6" plane through (0, 0.6, 0) normal (0, 1, 0) x (1, 0, 0)
  line L0 (-21.25, -37.5) -> (21.25, -37.5) projected
  line L1 (21.25, 37.5) -> (-21.25, 37.5) projected
  line L2 (-11.25, -37.5) -> (-0.4523, -18.7977)
  line L3 (-0.4523, -18.7977) -> (18.25, -37.5)
  line L4 (-18.25, 37.5) -> (0.4523, 18.7977)
  line L5 (0.4523, 18.7977) -> (11.25, 37.5)
  line L6 (-11.3137, 16.9706) -> (16.9706, -11.3137) projected
  line L7 (11.3137, -16.9706) -> (-16.9706, 11.3137) projected
  line L8 (-21.25, 37.5) -> (-21.25, -37.5) projected
  line L9 (21.25, -37.5) -> (21.25, 37.5) projected
  point P0 (0, 0)
  dimension "d26" = 10
  dimension "d27" = 3
  dimension "d28" = 3
  dimension "d29" = 10
  dimension "d30" = 60
  constraints: 8 end point, 4 parallel, 4 point on line
  measures "d26" distance from line of L8 L2.start
  measures "d27" distance from line of L9 L3.end
  measures "d28" distance from line of L8 L4.start
  measures "d29" distance of L1.start L5.end
  measures "d30" angle of L0 L2
extrude "押し出し5" cut sketch "スケッチ6" against normal through all contours L2 L3 L0 | L1 L5 L4
fillet "フィレット1" radius 5 2 edges at (-0.4523, 0, 18.7977) (0.4523, 0, -18.7977)
sketch "スケッチ7" plane through (0, 0, 0) normal (1, 0, 0) x (0, 1, 0)
  circle A0 centre (-3.4, 32.5) radius 1.75 projected
  circle A1 centre (-3.4, -32.5) radius 1.75 projected
  arc A2 (-4.535, 36.3356) -> (-4.535, 28.6644) centre (-3.4, 32.5) ccw projected
  line L0 (-3.4, 29.2668) -> (-6.2, 30.8834)
  line L1 (-6.2, 30.8834) -> (-6.2, 34.1166)
  line L2 (-6.2, 34.1166) -> (-3.4, 35.7332)
  line L3 (-3.4, 35.7332) -> (-0.6, 34.1166)
  line L4 (-0.6, 34.1166) -> (-0.6, 30.8834)
  line L5 (-0.6, 30.8834) -> (-3.4, 29.2668)
  line L6 (-3.4, -35.7332) -> (-6.2, -34.1166)
  line L7 (-6.2, -34.1166) -> (-6.2, -30.8834)
  line L8 (-6.2, -30.8834) -> (-3.4, -29.2668)
  line L9 (-3.4, -29.2668) -> (-0.6, -30.8834)
  line L10 (-0.6, -30.8834) -> (-0.6, -34.1166)
  line L11 (-0.6, -34.1166) -> (-3.4, -35.7332)
  point P0 (0, 0)
  dimension "d34" = 5.6
  dimension "d35" = 5.6
  constraints: 24 end point, 2 coincident, 2 vertical alignment, 26 other
  measures "d34" distance between parallel lines of L7 L10
  measures "d35" distance between parallel lines of L4 L1
extrude "押し出し6" cut sketch "スケッチ7" along normal mid plane 38
fillet "フィレット2" radius 2 4 edges at (-11.25, 0, 37.5) (18.25, 0, 37.5) (11.25, 0, -37.5) (-18.25, 0, -37.5)
equation "\"d5\" = d4"
equation "\"d7\" = d6"
equation "\"d9\" = d8"
equation "\"d28\" = d27"
equation "\"d29\" = d26"
equation "\"d35\" = d34"
